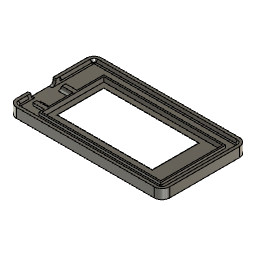
Soldered Inkplate 2 Case 3D (Autodesk Fusion 360 archive; units mm, degrees)
design "Inkplate 2 Top"
Autodesk Fusion 360 part; units mm, degrees
sketch "Sketch1" plane through (0, 0, 0) normal (0, 0, 1) x (1, 0, 0)
  line L0 (32.6, 17.6) -> (-32.6, 17.6)
  line L1 (-32.6, 17.6) -> (-32.6, -17.6)
  line L2 (-32.6, -17.6) -> (32.6, -17.6)
  line L3 (32.6, -17.6) -> (32.6, 17.6)
  line L4 (32.6, 17.6) -> (-32.6, -17.6) construction
  line L5 (-32.6, 17.6) -> (32.6, -17.6) construction
  line L6 (42.352, 22.1) -> (-37.1, 22.1)
  line L7 (-37.1, 22.1) -> (-37.1, -22.1)
  line L8 (-37.1, -22.1) -> (42.352, -22.1)
  line L9 (42.352, -22.1) -> (42.352, 22.1)
  line L10 (42.352, 22.1) -> (-37.1, -22.1) construction
  line L11 (-37.1, 22.1) -> (42.352, -22.1) construction
  line L12 (27.3, 12.1) -> (-22.048, 12.1)
  line L13 (-22.048, 12.1) -> (-22.048, -12.1)
  line L14 (-22.048, -12.1) -> (27.3, -12.1)
  line L15 (27.3, -12.1) -> (27.3, 12.1)
  line L16 (27.3, 12.1) -> (-22.048, -12.1) construction
  line L17 (-22.048, 12.1) -> (27.3, -12.1) construction
  point P0 (2.626, 0)
  point P1 (2.626, 0)
  dimension "d1" = 65.2
  dimension "d2" = 35.2
  dimension "d3" = 9.752
  dimension "d4" = 4.5
  dimension "d5" = 4.5
  dimension "d6" = 4.5
  dimension "d7" = 5.5
  dimension "d8" = 5.3
  constraint horizontal L0
  constraint perpendicular L0 L1
  constraint parallel L0 L2
  constraint parallel L1 L3
  constraint coincident L4 origin
  constraint coincident L5 origin
  constraint horizontal L6
  constraint vertical L7
  constraint horizontal L8
  constraint vertical L9
  constraint midpoint L11 P1
  constraint horizontal L12
  constraint perpendicular L12 L13
  constraint parallel L12 L14
  constraint parallel L13 L15
  constraint coincident L16 P1
  constraint coincident L17 P1
  constraint coincident P1 P0
  measures "d1" distance of L1.end L2.end
  measures "d2" distance of L0.end L1.end
  measures "d3" distance of L3 L9
  measures "d4" distance of L1 L7
  measures "d5" distance of L0 L6
  measures "d6" distance of L2 L8
  measures "d7" distance of L0 L12
  measures "d8" distance of L3 L15
extrude "Extrude1" add sketch "Sketch1" along normal blind 5 contours L0 L1 L2 L3 | L6 L7 L8 L9
sketch "Sketch2" plane through (0, 0, 5) normal (0, 0, 1) x (-1, 0, 0)
  line L0 (-27.3, -12.1) -> (-27.3, 12.1)
  line L1 (-27.3, 12.1) -> (22.048, 12.1)
  line L2 (22.048, 12.1) -> (22.048, -12.1)
  line L3 (22.048, -12.1) -> (-27.3, -12.1)
  line L4 (-42.352, 22.1) -> (-42.352, -22.1)
  line L5 (-42.352, -22.1) -> (37.1, -22.1)
  line L6 (37.1, -22.1) -> (37.1, 22.1)
  line L7 (37.1, 22.1) -> (-42.352, 22.1)
  line L8 (37.1, 22.1) -> (-42.352, -22.1) construction
  line L9 (-42.352, 22.1) -> (37.1, -22.1) construction
  line L10 (35.6, 20.6) -> (-40.852, 20.6)
  line L11 (-40.852, 20.6) -> (-40.852, -20.6)
  line L12 (-40.852, -20.6) -> (35.6, -20.6)
  line L13 (35.6, -20.6) -> (35.6, 20.6)
  line L14 (35.6, 20.6) -> (-40.852, -20.6) construction
  line L15 (-40.852, 20.6) -> (35.6, -20.6) construction
  point P0 (-2.626, 0)
  dimension "d11" = 1.5
  dimension "d12" = 1.5
  constraint coincident L6.end L7.start
  constraint coincident L4.end L5.start
  constraint coincident L4.start L7.end
  constraint coincident L5.end L6.start
  constraint horizontal L10
  constraint perpendicular L10 L11
  constraint parallel L10 L12
  constraint parallel L11 L13
  constraint coincident L14 P0
  constraint coincident L15 P0
  constraint midpoint L8 P0
  measures "d11" distance of L7 L10
  measures "d12" distance of L6 L13
extrude "Extrude2" cut sketch "Sketch2" against normal blind 3 contours L10 L11 L12 L13
sketch "Sketch3" plane through (0, 0, 2) normal (0, 0, 1) x (-1, 0, 0)
  line L0 (22.048, 12.1) -> (22.048, -12.1)
  line L1 (22.048, -12.1) -> (-27.3, -12.1)
  line L2 (-27.3, -12.1) -> (-27.3, 12.1)
  line L3 (-27.3, 12.1) -> (22.048, 12.1)
  line L4 (35.6, -20.6) -> (35.6, 20.6)
  line L5 (35.6, 20.6) -> (-40.852, 20.6)
  line L6 (-40.852, 20.6) -> (-40.852, -20.6)
  line L7 (-40.852, -20.6) -> (35.6, -20.6)
  line L8 (29, 12.1) -> (44, 12.1) construction
  line L9 (37.1, 22.1) -> (-42.352, 22.1)
  line L10 (24.748, 12.1) -> (26.748, 12.1)
  line L11 (26.748, 12.1) -> (26.748, -0.9)
  line L12 (26.748, -0.9) -> (24.748, -0.9)
  line L13 (24.748, -0.9) -> (24.748, 12.1)
  line L14 (22.048, 12.1) -> (-27.3, -12.1) construction
  line L15 (29.2, 14.8) -> (-34.452, 14.8)
  line L16 (-34.452, 14.8) -> (-34.452, -14.8)
  line L17 (-34.452, -14.8) -> (29.2, -14.8)
  line L18 (29.2, -14.8) -> (29.2, 14.8)
  line L19 (29.2, 14.8) -> (-34.452, -14.8) construction
  line L20 (-34.452, 14.8) -> (29.2, -14.8) construction
  line L21 (29.2, 14.8) -> (24.748, 14.8)
  line L22 (24.748, 14.8) -> (24.748, -14.8)
  line L23 (24.748, -14.8) -> (29.2, -14.8)
  line L24 (29.2, -14.8) -> (29.2, 14.8)
  line L25 (24.748, -0.9) -> (35.6, -0.9)
  line L26 (35.6, -0.9) -> (35.6, -2.9)
  line L27 (35.6, -2.9) -> (24.748, -2.9)
  line L28 (24.748, -2.9) -> (24.748, -0.9)
  line L29 (24.748, 12.1) -> (35.6, 12.1)
  line L30 (35.6, 12.1) -> (35.6, 14.1)
  line L31 (35.6, 14.1) -> (24.748, 14.1)
  line L32 (24.748, 14.1) -> (24.748, 12.1)
  line L33 (32.6, 28) -> (32.6, -11)
  line L34 (37.1, -22.1) -> (37.1, 22.1)
  line L35 (-36.452, 16.8) -> (26.748, 16.8)
  line L36 (26.748, 16.8) -> (26.748, -16.8)
  line L37 (26.748, -16.8) -> (-36.452, -16.8)
  line L38 (-36.452, -16.8) -> (-36.452, 16.8)
  point P0 (-2.626, 0)
  dimension "d15" = 10
  dimension "d16" = 2
  dimension "d17" = 13
  dimension "d19" = 2.7
  dimension "d20" = 59.2
  dimension "d21" = 2
  dimension "d22" = 2
  dimension "d34" = 4.5
  dimension "d35" = 2.7
  dimension "d36" = 2
  dimension "d37" = 2
  dimension "d38" = 2
  dimension "d39" = 2
  constraint horizontal L8
  constraint horizontal L10
  constraint vertical L11
  constraint horizontal L12
  constraint vertical L13
  constraint coincident L8 L10.start
  constraint coincident L0.start L3.end
  constraint coincident L1.end L2.start
  constraint horizontal L15
  constraint perpendicular L15 L16
  constraint parallel L15 L17
  constraint parallel L16 L18
  constraint coincident L19 P0
  constraint coincident L20 P0
  constraint midpoint L14 P0
  constraint horizontal L21
  constraint vertical L22
  constraint horizontal L23
  constraint vertical L24
  constraint coincident L17 L18.start
  constraint coincident L10.start L22
  constraint horizontal L25
  constraint vertical L26
  constraint horizontal L27
  constraint vertical L28
  constraint coincident L4 L26.end
  constraint horizontal L29
  constraint vertical L30
  constraint horizontal L31
  constraint vertical L32
  constraint coincident L4 L30.end
  constraint perpendicular L9 L33
  constraint horizontal L35
  constraint vertical L36
  constraint horizontal L37
  constraint vertical L38
  measures "d15" distance of L8 L9
  measures "d16" distance of L10.start L10.end
  measures "d17" distance of L10.start L12.end
  measures "d19" distance of L3 L15
  measures "d20" distance of L16 L22
  measures "d21" distance of L25 L27
  measures "d22" distance of L10.start L31.end
  measures "d34" distance of L33 L34
  measures "d35" distance of L0 L22
  measures "d36" distance of L22 L36
  measures "d37" distance of L17 L37
  measures "d38" distance of L16 L38
  measures "d39" distance of L15 L35
extrude "Extrude3" add sketch "Sketch3" along normal blind 1.3 contours L18 L24 L25 L27 L33 | L18 L24 L25 L27 L36 | L18 L24 L29 L31 L33 | L12 L22 L25 L27 L28 L36 | L18 L24 L29 L31 L36 | L10 L11 L12 L13 L22 L25 L29 L36 | L10 L22 L29 L31 L32 L36
sketch "Sketch4" plane through (-37.1, 0, 0) normal (-1, 0, 0) x (0, -1, 0)
  line L0 (-22.1, 0) -> (22.1, 0)
  line L1 (22.1, 0) -> (22.1, 5)
  line L2 (22.1, 5) -> (-22.1, 5)
  line L3 (-22.1, 5) -> (-22.1, 0)
  line L4 (12.1, 5) -> (-0.9, 5)
  line L5 (-0.9, 5) -> (-0.9, 2)
  line L6 (-0.9, 2) -> (12.1, 2)
  line L7 (12.1, 2) -> (12.1, 5)
  dimension "d25" = 13
  dimension "d26" = 3
  dimension "d27" = 10
  constraint horizontal L4
  constraint vertical L5
  constraint horizontal L6
  constraint vertical L7
  constraint coincident L2 L4.start
  measures "d25" distance of L4.start L4.end
  measures "d26" distance of L4.start L6.end
  measures "d27" distance of L1 L7
extrude "Extrude4" cut sketch "Sketch4" against normal blind 6 contours L2 L4 L5 L6 L7
fillet "Fillet1" radius 2 4 edges at (-29.674, -12.1, 2) (-29.674, 0.9, 2) (-36.35, -12.1, 2) (-36.35, 0.9, 2)
fillet "Fillet2" radius 4 4 edges at (-37.1, 22.1, 2.5) (-37.1, -22.1, 2.5) (42.352, -22.1, 2.5) (42.352, 22.1, 2.5)
extrude "Extrude5" add sketch "Sketch3" along normal blind 1.3 contours L17 L22 L23 L27 L36 | L15 L16 L17 L21 L23 L35 L36 L37 L38 | L15 L21 L22 L31 L36
extrude "Extrude7" add 1 faces at (32.068, -4.0333, 2) along direction (0, 0, 1) blind 0.1
chamfer "Chamfer1" distance 1.2 angle 45 4 edges at (4.852, -14.8, 3.3) (-24.748, 0, 3.3) (4.852, 14.8, 3.3) (34.452, 0, 3.3)
ref_plane "WorkPlane1" through (1.876, 0, 2.5) normal (0, 0, 1) x (1, 0, 0)
sketch "Sketch5" plane through (1.876, 0, 2.5) normal (0, 0, 1) x (1, 0, 0)
  line L0 (-42, 2.9) -> (-23, 2.9) construction
  line L1 (-34.476, -14.1) -> (-41.7772, -14.1) construction
  line L2 (-37.476, 2.9) -> (-36.476, 2.9)
  line L3 (-36.476, 2.9) -> (-36.476, 18.6)
  line L4 (-36.476, 20.6) -> (-37.476, 20.6)
  line L5 (-37.476, 20.6) -> (-37.476, 2.9)
  line L6 (-37.476, 0.9) -> (-37.476, 20.6)
  line L7 (-37.476, 20.6) -> (38.976, 20.6)
  line L8 (-37.476, 20.6) -> (38.976, 20.6)
  line L9 (38.976, 20.6) -> (38.976, 19.6)
  line L10 (36.976, 19.6) -> (-35.476, 19.6)
  line L11 (-37.476, 19.6) -> (-37.476, 20.6)
  line L12 (38.976, 20.6) -> (38.976, -20.6)
  line L13 (38.976, 20.6) -> (37.976, 20.6)
  line L14 (37.976, 18.6) -> (37.976, -18.6)
  line L15 (37.976, -20.6) -> (38.976, -20.6)
  line L16 (38.976, -20.6) -> (38.976, 20.6)
  line L17 (38.976, -20.6) -> (-37.476, -20.6)
  line L18 (38.976, -20.6) -> (-37.476, -20.6)
  line L19 (-37.476, -20.6) -> (-37.476, -19.6)
  line L20 (-35.476, -19.6) -> (36.976, -19.6)
  line L21 (38.976, -19.6) -> (38.976, -20.6)
  line L22 (-37.476, -20.6) -> (-37.476, -12.1)
  line L23 (-37.476, -20.6) -> (-36.476, -20.6)
  line L24 (-36.476, -18.6) -> (-36.476, -14.1)
  line L25 (-36.476, -14.1) -> (-37.476, -14.1)
  line L26 (-37.476, -14.1) -> (-37.476, -20.6)
  arc A0 (-35.476, 19.6) -> (-36.476, 18.6) centre (-35.476, 18.6) ccw
  arc A1 (37.976, 18.6) -> (36.976, 19.6) centre (36.976, 18.6) ccw
  arc A2 (36.976, -19.6) -> (37.976, -18.6) centre (36.976, -18.6) ccw
  arc A3 (-36.476, -18.6) -> (-35.476, -19.6) centre (-35.476, -18.6) ccw
  point P0 (-34.476, 2.9)
  point P1 (-34.476, -14.1)
  dimension "d44" = 1
  dimension "d45" = 1
  dimension "d46" = 1
  dimension "d47" = 1
  dimension "d48" = 1
  dimension "d49" = 1
  constraint horizontal L0
  constraint horizontal L1
  constraint horizontal L2
  constraint vertical L3
  constraint horizontal L4
  constraint vertical L5
  constraint coincident L0 L2.start
  constraint coincident L2.start L6
  constraint coincident L4.start L7
  constraint horizontal L8
  constraint vertical L9
  constraint horizontal L10
  constraint vertical L11
  constraint coincident L4.end L5.start
  constraint coincident L9.end L12
  constraint horizontal L13
  constraint vertical L14
  constraint horizontal L15
  constraint vertical L16
  constraint coincident L7.end L8.end
  constraint coincident L15.start L17
  constraint horizontal L18
  constraint vertical L19
  constraint horizontal L20
  constraint vertical L21
  constraint coincident L12.end L15.end
  constraint coincident L19.end L22
  constraint horizontal L23
  constraint vertical L24
  constraint horizontal L25
  constraint vertical L26
  constraint coincident L17.end L18.end
  constraint coincident L1 L24.end
  constraint coincident L11.start L10
  constraint coincident L4.start L3
  constraint tangent L10 A0
  constraint tangent L3 A0
  constraint coincident L13.end L14
  constraint coincident L9.end L10
  constraint tangent L14 A1
  constraint tangent L10 A1
  constraint equal A0 A1
  constraint coincident L15.start L14
  constraint coincident L21.start L20
  constraint tangent L14 A2
  constraint tangent L20 A2
  constraint equal A0 A2
  constraint coincident L23.end L24
  constraint coincident L19.end L20
  constraint tangent L24 A3
  constraint tangent L20 A3
  constraint equal A0 A3
  measures "d44" distance of L2.start L2.end
  measures "d45" distance of L4.end L11.start
  measures "d46" distance of L7.end L13.end
  measures "d47" distance of L12.end L21.start
  measures "d48" distance of L17.end L23.end
  measures "d49" radius of A0
extrude "Extrude6" add sketch "Sketch5" along normal blind 2.5
chamfer "Chamfer2" distance 1.5 angle 45 9 edges at (-34.6, 10.75, 2.5) (-34.3071, 19.3071, 2.5) (2.626, 19.6, 2.5) (39.5591, 19.3071, 2.5) (39.852, 0, 2.5) (39.5591, -19.3071, 2.5) (2.626, -19.6, 2.5) (-34.3071, -19.3071, 2.5) (-34.6, -16.35, 2.5)
chamfer "Chamfer3" distance 1 angle 45 9 edges at (-34.6, 10.75, 5) (-34.3071, 19.3071, 5) (2.626, 19.6, 5) (39.5591, 19.3071, 5) (39.852, 0, 5) (39.5591, -19.3071, 5) (2.626, -19.6, 5) (-34.3071, -19.3071, 5) (-34.6, -16.35, 5)
chamfer "Chamfer4" distance 2 angle 45 4 edges at (2.626, -12.1, 0) (-22.048, 0, 0) (27.3, 0, 0) (2.626, 12.1, 0)
